Autodesk Fusion 360 part; units mm, degrees
(part 2 of 2)
sketch "Sketch1" plane through (0, 0, 0) normal (0, 1, 0) x (1, 0, 0)
  line L0 (0, 0) -> (-48, 0) construction
  line L1 (-48, 0) -> (-68, 0) construction
  line L2 (0, 0) -> (0, 52) construction
  line L3 (-9.7468, 47) -> (-68, 47)
  line L4 (-68, 47) -> (-68, 0) construction
  line L5 (-45.1052, -16.417) -> (-31.4244, -54.0047)
  line L6 (-53.4275, -54.0047) -> (-68, -54.0047) construction
  line L7 (-68, -54.0047) -> (-68, 0) construction
  line L8 (-53.4275, -54.0047) -> (-68, -13.967)
  line L9 (-100, 35.633) -> (-100, 30.833) construction
  line L10 (-100, 30.833) -> (0, 30.833) construction
  line L11 (0, 0) -> (0, -9.167) construction
  line L12 (0, -9.167) -> (-100, -9.167) construction
  line L13 (-100, -9.167) -> (-100, -13.967) construction
  line L14 (0, -13.967) -> (0, -9.167) construction
  line L15 (-100, -9.167) -> (-100, 30.833) construction
  arc A0 (-9.7468, 47) -> (-45.1052, -16.417) centre (0, 0) ccw
  arc A1 (-45.1052, -16.417) -> (0, 48) centre (0, 0) ccw construction
  arc A2 (0, 48) -> (-9.7468, 47) centre (0, 0) ccw construction
  line L16 (-31.4244, -54.0047) -> (-53.4275, -54.0047)
  line L17 (-63.2, 35.633) -> (-63.2, -13.967)
  line L18 (0, 35.633) -> (-63.2, 35.633) construction
  line L19 (-68, 35.633) -> (-100, 35.633) construction
  line L20 (-65.3213, 35.633) -> (-68, 35.633)
  line L21 (-68, 47) -> (-68, 35.633)
  line L22 (-100, -13.967) -> (-68, -13.967) construction
  line L23 (-63.2, -13.967) -> (0, -13.967) construction
  line L24 (-68, -13.967) -> (-65.3213, -13.967)
  line L25 (0, 0) -> (-40, 42) construction
  line L26 (-40, 42) -> (-40, 47) construction
  circle A3 centre (-40, 42) radius 1.5
  circle A4 centre (-56, 42) radius 1.5
  line L27 (0, 0) -> (-55.8448, -4.167) construction
  line L28 (-55.8448, -4.167) -> (-55.8448, -9.167) construction
  circle A5 centre (-55.8448, -4.167) radius 1.5
  line L29 (-100, 10.833) -> (-63.2, 10.833) construction
  line L30 (-63.2, 10.833) -> (-55.2, 10.833) construction
  line L31 (-55.2, 9.333) -> (-55.2, 12.333) construction
  line L32 (-64.2607, -12.9063) -> (-63.2, -13.967) construction
  arc A6 (-65.3213, -13.967) -> (-63.2, -11.8457) centre (-64.2607, -12.9063) ccw
  arc A7 (-63.2, -11.8457) -> (-65.3213, -13.967) centre (-64.2607, -12.9063) ccw construction
  line L33 (-65.3213, -13.967) -> (-63.2, -13.967) construction
  line L34 (-63.2, 35.633) -> (-64.2607, 34.5723) construction
  arc A8 (-63.2, 33.5117) -> (-65.3213, 35.633) centre (-64.2607, 34.5723) ccw
  arc A9 (-65.3213, 35.633) -> (-63.2, 33.5117) centre (-64.2607, 34.5723) ccw construction
  line L35 (-63.2, 35.633) -> (-65.3213, 35.633) construction
  point P0 (-68, -13.967)
  point P1 (-33.1034, 34.7586)
  point P2 (-47.8669, -3.5717)
  point P3 (-100, 10.833)
  point P4 (-55.2, 10.833)
  dimension "d1" = 96
  dimension "d2" = 20
  dimension "d3" = 52
  dimension "d4" = 5
  dimension "d5" = 40
  dimension "d6" = 70
  dimension "d8" = 4.8
  dimension "d9" = 16.367
  dimension "d10" = 100
  dimension "d11" = 4.8
  dimension "d12" = 40
  dimension "d14" = 4.8
  dimension "d15" = 5
  dimension "d16" = 10
  dimension "d17" = 3
  dimension "d18" = 3
  dimension "d19" = 12
  dimension "d20" = 5
  dimension "d21" = 8
  dimension "d22" = 5
  dimension "d23" = 3
  dimension "d24" = 8
  dimension "d25" = 3
  dimension "d43" = 3
  dimension "d44" = 1.5
  dimension "d45" = 45
  dimension "d46" = 1.5
  dimension "d47" = 45
  constraint coincident L0.start L2.start
  constraint coincident L0.end A0
  constraint horizontal L0
  constraint parallel L0 L1
  constraint perpendicular L0 L2
  constraint parallel L1 L3
  constraint perpendicular L1 L4
  constraint tangent L5 A0
  constraint perpendicular L4 L6
  constraint perpendicular L1 L7
  constraint coincident L7 P0
  constraint parallel L5 L8
  constraint coincident L2 L18.start
  constraint perpendicular L2 L18
  constraint perpendicular L9 L18
  constraint coincident L2 L10.end
  constraint perpendicular L2 L10
  constraint perpendicular L0 L11
  constraint perpendicular L9 L12
  constraint perpendicular L12 L13
  constraint perpendicular L13 L22
  constraint perpendicular L12 L14
  constraint perpendicular L10 L15
  constraint coincident P0 L22
  constraint coincident L8 P0
  constraint coincident L2 A1.end
  constraint concentric A0 A1
  constraint concentric A0 A2
  constraint perpendicular L4 L16
  constraint coincident L17.start L18.end
  constraint coincident L17.end L22
  constraint perpendicular L17 L22
  constraint coincident L4 L19.start
  constraint parallel L10 L19
  constraint collinear L18 L20
  constraint collinear L23 L24
  constraint coincident L3 L26.end
  constraint perpendicular L3 L26
  constraint coincident L25 P1
  constraint coincident A0 P1
  constraint coincident L25.end L26.start
  constraint coincident L12 L28.end
  constraint perpendicular L12 L28
  constraint coincident A0 P2
  constraint coincident L27 P2
  constraint coincident L27.end L28.start
  constraint midpoint L15 P3
  constraint coincident P3 L29.start
  constraint midpoint L17 L29.end
  constraint perpendicular L17 L30
  constraint perpendicular L30 L31
  constraint midpoint L31 P4
  constraint coincident P4 L30.end
  constraint coincident L32.start A6.centre
  constraint coincident L17 A6.end
  constraint concentric A6 A7
  constraint collinear L23 L33
  constraint coincident L34.end A8.centre
  constraint coincident L17.start A8
  constraint coincident L17 A8.start
  constraint concentric A8 A9
  constraint collinear L18 L35
  measures "d1" diameter of A0
  measures "d2" distance of L0.end L1.end
  measures "d3" distance of L0.start L2.end
  measures "d4" distance of L2.end L3
  measures "d5" distance of L5.start L5.end
  measures "d6" angle of L0 L5
  measures "d8" distance of L9.start L9.end
  measures "d9" distance of L2.end L18
  measures "d10" distance of L18.start L9.start
  measures "d11" distance of L12.end L13.end
  measures "d12" distance of L9.end L12.end
  measures "d14" distance of L4 L17.start
  measures "d15" distance of L25.end L26.end
  measures "d16" distance of L25.end P1
  measures "d17" diameter of A3
  measures "d18" diameter of A4
  measures "d19" distance of L4 A4.centre
  measures "d20" distance of L3 A4.centre
  measures "d21" distance of L27.end P2
  measures "d22" distance of L27.end L28.end
  measures "d23" diameter of A5
  measures "d24" distance of L29.end P4
  measures "d25" distance of L31.start L31.end
  measures "d43" diameter of A6
  measures "d44" distance of L17.end L32.start
  measures "d45" angle of L24 L32
  measures "d46" distance of L17.start L34.end
  measures "d47" angle of L20 L34
extrude "Extrude1" add sketch "Sketch1" along normal blind 4.8 contours L3 L5 L8 A0 L16 L17 L20 L21 L24 A6 A8
sketch "Sketch2" plane through (-63.2, 0, 0) normal (-1, 0, 0) x (0, -1, 0)
  line L0 (0, -33.5117) -> (0, 11.8457)
  line L1 (-4.8, 11.8457) -> (-4.8, -33.5117)
  line L2 (0, -10.833) -> (-2.4, -10.833) construction
  circle A0 centre (-2.4, -10.833) radius 1.5
  line L3 (0, 11.8457) -> (-4.8, 11.8457)
  line L4 (-4.8, -33.5117) -> (0, -33.5117)
  point P0 (0, -10.833)
  dimension "d35" = 2.4
  dimension "d36" = 3
  constraint coincident P0 L2.start
  constraint perpendicular L0 L2
  constraint coincident L2.end A0.centre
  measures "d35" distance of P0 L2.end
  measures "d36" diameter of A0
extrude "Extrude2" cut sketch "Sketch2" against normal blind 8 contours A0
fillet "Fillet1" radius 4 1 edges at (-68, 2.4, -47)
fillet "Fillet1" radius 4 1 edges at (-53.4275, 2.4, 54.0047)
thread "Thread1" "ISO Metric profile 3.0 M3x0.5 6H" major diameter 3.086 minor diameter 2.529 pitch 0.5 angle 60 resizes the face on face at (-60.5333, 0.9075, -10.9824)
sketch "Sketch3" plane through (0, 0, 0) normal (0, -1, 0) x (1, 0, 0)
  circle A0 centre (-55.8448, 4.167) radius 1.5
  circle A1 centre (-56, -42) radius 1.5
  circle A2 centre (-40, -42) radius 1.5
  arc A3 (-45.1052, 16.417) -> (-9.7468, -47) centre (0, 0) ccw
  line L0 (-45.1052, 16.417) -> (-31.4244, 54.0047)
  line L1 (-31.4244, 54.0047) -> (-50.6266, 54.0047)
  arc A4 (-50.6266, 54.0047) -> (-54.3854, 51.3728) centre (-50.6266, 50.0047) ccw
  line L2 (-54.3854, 51.3728) -> (-68, 13.967)
  line L3 (-68, 13.967) -> (-65.3213, 13.967)
  arc A5 (-63.2, 11.8457) -> (-65.3213, 13.967) centre (-64.2607, 12.9063) ccw
  line L4 (-63.2, 11.8457) -> (-63.2, -33.5117)
  arc A6 (-65.3213, -35.633) -> (-63.2, -33.5117) centre (-64.2607, -34.5723) ccw
  line L5 (-65.3213, -35.633) -> (-68, -35.633)
  line L6 (-68, -35.633) -> (-68, -43)
  arc A7 (-68, -43) -> (-64, -47) centre (-64, -43) ccw
  line L7 (-64, -47) -> (-9.7468, -47)
  arc A8 (-45.1052, 16.417) -> (-9.7468, -47) centre (0, 0) ccw
  line L8 (-9.7468, -47) -> (-68, -47)
  line L9 (-45.1052, 16.417) -> (-31.4244, 54.0047)
  arc A9 (-49.8037, 18.1271) -> (-24.4949, -47) centre (0, 0) ccw
  arc A10 (-24.4949, -47) -> (-37.4193, 37.5339) centre (0, 0) ccw construction
  line L10 (-49.8037, 18.1271) -> (-44.3442, 33.1271)
  line L11 (-63.2, 13.967) -> (0, 13.967)
  line L12 (-44.3442, 33.1271) -> (-59.6259, 33.1271)
  line L13 (-61.0263, 33.1271) -> (-54.3854, 51.3728)
  line L14 (-50.6266, 54.0047) -> (-31.4244, 54.0047)
  line L15 (-31.4244, 54.0047) -> (-45.1052, 16.417)
  arc A11 (-50.6266, 54.0047) -> (-54.3854, 51.3728) centre (-50.6266, 50.0047) ccw
  arc A12 (-50.6266, 54.0047) -> (-54.3854, 51.3728) centre (-50.6266, 50.0047) ccw
  arc A13 (-54.3854, 51.3728) -> (-50.6266, 54.0047) centre (-50.6266, 50.0047) ccw construction
  line L16 (-53.4275, 54.0047) -> (-68, 13.967)
  arc A14 (-59.6259, 33.1271) -> (-61.5053, 31.8111) centre (-59.6259, 31.1271) ccw
  arc A15 (-61.5053, 31.8111) -> (-59.6259, 33.1271) centre (-59.6259, 31.1271) ccw construction
  line L17 (-59.6259, 33.1271) -> (-61.0263, 33.1271) construction
  line L18 (-61.0263, 33.1271) -> (-61.5053, 31.8111)
  arc A16 (-45.1052, 16.417) -> (-9.7468, -47) centre (0, 0) ccw
  arc A17 (-45.1052, 16.417) -> (-9.7468, -47) centre (0, 0) ccw
  line L19 (-24.4949, -47) -> (-9.7468, -47)
  arc A18 (-37.4193, 37.5339) -> (-49.8037, 18.1271) centre (0, 0) ccw construction
  dimension "d51" = 106
  dimension "d52" = 70
  dimension "d53" = 15
  dimension "d54" = 4
  dimension "d55" = 48
  constraint concentric A3 A9
  constraint coincident L7 A9.end
  constraint coincident L0 A10.end
  constraint concentric A9 A10
  constraint tangent A9 L10
  constraint coincident L2 L13.start
  constraint horizontal L12
  constraint coincident A4.end L2.start
  constraint coincident L1.end A4.start
  constraint coincident L0.end L1.start
  constraint coincident A3.start L0.start
  constraint concentric A4 A12
  constraint concentric A12 A13
  constraint tangent L12 A14
  constraint tangent L16 A14
  constraint coincident L2 A14.end
  constraint concentric A14 A15
  constraint horizontal L17
  constraint coincident A3.end L7.end
  constraint concentric A9 A18
  measures "d51" diameter of A9
  measures "d52" angle of L10 L11
  measures "d53" vertical distance of A9.start L10.end
  measures "d54" diameter of A14
  measures "d55" radius of A17
extrude "Extrude3" cut sketch "Sketch3" against normal through all contours A3 L0 L1 A4 L2 A8 L9 A9 L10 L11 L12 L13 L14 L15 A11 A12 L16 A14 L18 A16 A17 | A3 L7 A8 L8 A9 L11 A16 A17 L19
thread "Thread2" "ISO Metric profile 3.0 M3x0.5 6H" major diameter 3.086 minor diameter 2.529 pitch 0.5 angle 60 resizes the face on face at (-54.3466, 1.6, 4.0922)
thread "Thread3" "ISO Metric profile 3.0 M3x0.5 6H" major diameter 3.086 minor diameter 2.529 pitch 0.5 angle 60 resizes the face on face at (-57.4095, 3.2, -42.513)
thread "Thread4" "ISO Metric profile 3.0 M3x0.5 6H" major diameter 3.086 minor diameter 2.529 pitch 0.5 angle 60 resizes the face on face at (-38.5905, 1.6, -42.513)
fillet "Fillet3" radius 1 1 edges at (-24.4949, 2.4, -47)
sketch "Sketch4" plane through (0, 0, 0) normal (0, -1, 0) x (1, 0, 0)
  arc A0 (-28.2843, -47) -> (-27.7605, -45.1481) centre (-28.2843, -46) ccw
  arc A1 (-49.8037, 18.1271) -> (-27.7605, -45.1481) centre (0, 0) ccw
  line L0 (-49.8037, 18.1271) -> (-44.3442, 33.1271)
  line L1 (-44.3442, 33.1271) -> (-59.6259, 33.1271)
  arc A2 (-59.6259, 33.1271) -> (-61.5053, 31.8111) centre (-59.6259, 31.1271) ccw
  line L2 (-61.5053, 31.8111) -> (-68, 13.967)
  line L3 (-68, 13.967) -> (-65.3213, 13.967)
  arc A3 (-63.2, 11.8457) -> (-65.3213, 13.967) centre (-64.2607, 12.9063) ccw
  line L4 (-63.2, 11.8457) -> (-63.2, -33.5117)
  arc A4 (-65.3213, -35.633) -> (-63.2, -33.5117) centre (-64.2607, -34.5723) ccw
  line L5 (-65.3213, -35.633) -> (-68, -35.633)
  line L6 (-68, -35.633) -> (-68, -43)
  arc A5 (-68, -43) -> (-64, -47) centre (-64, -43) ccw
  line L7 (-64, -47) -> (-28.2843, -47)
  circle A6 centre (-56.866, 9.347) radius 1.5
  line L8 (-56.866, 9.347) -> (-56.866, 24.347) construction
  arc A7 (-56.866, 24.347) -> (-58.1733, 24.2899) centre (-56.866, 9.347) ccw construction
  line L9 (-56.866, 9.347) -> (-56.866, 24.347) construction
  line L10 (-56.866, 9.347) -> (-58.1733, 24.2899) construction
  line L11 (-56.866, 24.347) -> (-56.866, 25.847) construction
  line L12 (-58.1733, 24.2899) -> (-58.3041, 25.7842) construction
  arc A8 (-56.866, 25.847) -> (-56.866, 22.847) centre (-56.866, 24.347) ccw construction
  arc A9 (-56.866, 22.847) -> (-56.866, 25.847) centre (-56.866, 24.347) ccw
  arc A10 (-58.0426, 22.7956) -> (-58.3041, 25.7842) centre (-58.1733, 24.2899) ccw construction
  arc A11 (-58.3041, 25.7842) -> (-58.0426, 22.7956) centre (-58.1733, 24.2899) ccw
  arc A12 (-56.866, 22.847) -> (-58.0426, 22.7956) centre (-56.866, 9.347) ccw
  arc A13 (-56.866, 25.847) -> (-58.3041, 25.7842) centre (-56.866, 9.347) ccw
  circle A14 centre (-55.8448, 4.167) radius 1.2645
  circle A15 centre (-56, -42) radius 1.2645
  circle A16 centre (-40, -42) radius 1.2645
  point P0 (-58.3041, 25.7842)
  point P1 (-56.866, 25.847)
  dimension "d59" = 3
  dimension "d60" = 56.866
  dimension "d61" = 9.347
  dimension "d62" = 15
  dimension "d63" = 3
  dimension "d64" = 5
  dimension "d65" = 3
  dimension "d66" = 13.5
  constraint coincident A6.centre L8.start
  constraint vertical L8
  constraint coincident L8.end A7.start
  constraint coincident A7.end L10.end
  constraint parallel L8 L11
  constraint parallel L10 L12
  constraint coincident P0 L12.end
  constraint coincident P1 L11.end
  constraint coincident L8 A8.end
  constraint coincident L10 A10.start
  constraint concentric A8 A9
  constraint concentric A10 A11
  constraint tangent A8 A13
  constraint tangent A9 A13
  measures "d59" diameter of A6
  measures "d60" horizontal distance of A6.centre A1.centre
  measures "d61" vertical distance of A6.centre A1.centre
  measures "d62" distance of A6.centre L8.end
  measures "d63" diameter of A8
  measures "d64" angle of L9 L10
  measures "d65" diameter of A10
  measures "d66" radius of A12
extrude "Extrude4" cut sketch "Sketch4" against normal through all contours A6 | A9 A11 A12 A13
thread "Thread5" "ISO Metric profile 3.0 M3x0.5 6H" major diameter 3.086 minor diameter 2.529 pitch 0.5 angle 60 resizes the face on face at (-55.3735, 1.6, 9.1976)

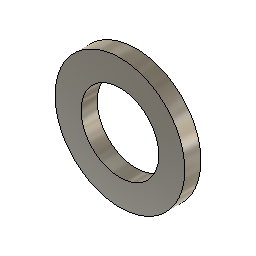
design "WasherM5"
Autodesk Fusion 360 part; units mm, degrees
sketch "Sketch1" plane through (0, 0, 0) normal (0, 1, 0) x (1, 0, 0)
  circle A0 centre (0, 0) radius 2.65
  circle A1 centre (0, 0) radius 4.425
  dimension "d1" = 5.3
  dimension "d2" = 8.85
  constraint coincident A0.centre A1.centre
  measures "d1" diameter of A0
  measures "d2" diameter of A1
extrude "Extrude1" add sketch "Sketch1" along normal blind 1.1

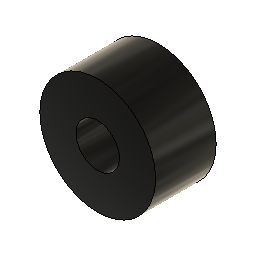
design "RampSpacer"
Autodesk Fusion 360 part; units mm, degrees
sketch "Sketch1" plane through (0, 0, 0) normal (0, 1, 0) x (1, 0, 0)
  circle A0 centre (0, 0) radius 1.5
  circle A1 centre (0, 0) radius 4
  dimension "d1" = 3
  dimension "d2" = 8
  constraint coincident A0.centre A1.centre
  constraint concentric A0 A1
  measures "d1" diameter of A0
  measures "d2" diameter of A1
extrude "Extrude1" add sketch "Sketch1" along normal blind 4.2

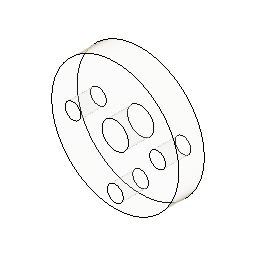
design "StatorSpacer"
Autodesk Fusion 360 part; units mm, degrees
sketch "Sketch1" plane through (0, 0, 0) normal (0, 1, 0) x (1, 0, 0)
  circle A0 centre (0, 0) radius 12
  circle A1 centre (0, 0) radius 9.5 construction
  circle A2 centre (0, 0) radius 8 construction
  line L0 (0, 0) -> (0, -9.5) construction
  line L1 (0, 0) -> (0, 9.5) construction
  line L2 (0, 0) -> (8, 0) construction
  line L3 (0, 0) -> (-8, 0) construction
  circle A3 centre (0, 9.5) radius 1.5
  circle A4 centre (8, 0) radius 1.5
  circle A5 centre (-8, 0) radius 1.5
  circle A6 centre (0, 0) radius 2.5
  dimension "d1" = 24
  dimension "d2" = 19
  dimension "d3" = 16
  dimension "d5" = 3
  dimension "d6" = 3
  dimension "d7" = 3
  dimension "d10" = 5
  constraint coincident A0.centre A1.centre
  constraint concentric A0 A1
  constraint coincident A1 L0.end
  constraint vertical L0
  constraint coincident A1 L1.end
  constraint parallel L0 L1
  constraint coincident A2 L2.end
  constraint perpendicular L0 L2
  constraint coincident A2 L3.end
  constraint perpendicular L0 L3
  constraint coincident L1.end A3.centre
  constraint coincident L2.end A4.centre
  constraint coincident L3.end A5.centre
  constraint concentric A0 A6
  measures "d1" diameter of A0
  measures "d2" diameter of A1
  measures "d3" diameter of A2
  measures "d5" diameter of A3
  measures "d6" diameter of A4
  measures "d7" diameter of A5
  measures "d10" diameter of A6
extrude "Extrude1" add sketch "Sketch1" along normal blind 4.8

design "Spacer M3x45"
Autodesk Fusion 360 part; units mm, degrees
sketch "Sketch1" plane through (0, 0, 0) normal (0, 1, 0) x (1, 0, 0)
  line L0 (2.725, 1.5733) -> (0, 3.1466)
  line L1 (0, 3.1466) -> (-2.725, 1.5733)
  line L2 (-2.725, 1.5733) -> (-2.725, -1.5733)
  line L3 (-2.725, -1.5733) -> (0, -3.1466)
  line L4 (0, -3.1466) -> (2.725, -1.5733)
  line L5 (2.725, -1.5733) -> (2.725, 1.5733)
  circle A0 centre (0, 0) radius 1.25
  dimension "d1" = 2.5
  measures "d1" diameter of A0
extrude "Extrude1" add sketch "Sketch1" along normal blind 45
